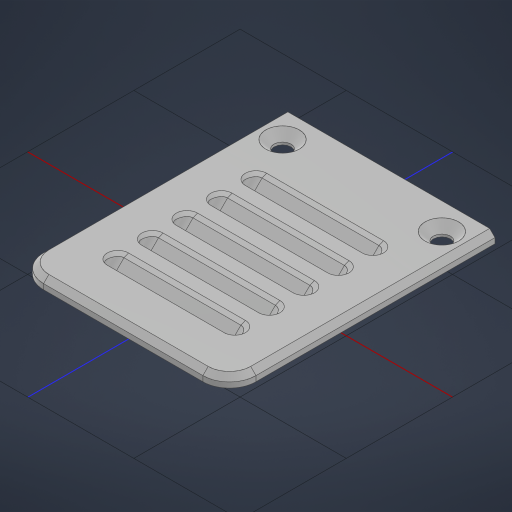
# Autodesk Inventor part: LED-Ring_Camera-Cover
Saved by Autodesk Inventor 2023.2 (Build 272271030, 271C)
## iProperties
Created: 2023-02-19
Part Number: LED-Ring_Camera-Cover
Material: Generisch
Document SubType Name: Modeling
Designer: Stefan
Mass: 3.244 g
Surface Area: 44.6567 cm^2
Volume: 3.244 cm^3
Density: 1 g/cm^3
Appearance: Glatt - Mittelgrau
Author: Stefan
Autodesk Inventor part; units mm, degrees
ref_plane "YZ Plane" through (0, 0, 0) normal (1, 0, 0) x (0, 1, 0)
ref_plane "XZ Plane" through (0, 0, 0) normal (0, 1, 0) x (-1, 0, 0)
ref_plane "XY Plane" through (0, 0, 0) normal (0, 0, 1) x (1, 0, 0)
sketch "Skizze1" plane through (0, 0, 0) normal (0, 1, 0) x (-1, 0, 0)
  arc A0 (20, 17) -> (15, 22) centre (15, 17) ccw
  arc A1 (-15, 22) -> (-20, 17) centre (-15, 17) ccw
  line L0 (20, -40) -> (-20, -40) construction
  line L1 (-20, -40) -> (-20, 22) construction
  line L2 (-20, 22) -> (20, 22) construction
  line L3 (20, 22) -> (20, -40) construction
  line L4 (20, -40) -> (-20, -40)
  line L5 (15, 22) -> (-15, 22)
  line L6 (20, -40) -> (20, 17)
  line L7 (-20, 17) -> (-20, -40)
  line L8 (0, -40) -> (0, 22) construction
  arc A2 (18, 17) -> (15, 20) centre (15, 17) ccw construction
  arc A3 (-15, 20) -> (-18, 17) centre (-15, 17) ccw construction
  line L9 (-15, 20) -> (15, 20) construction
  line L10 (20, -28) -> (-20, -28)
  line L11 (-20, -28) -> (-20, -26)
  line L12 (20, -26) -> (20, -28)
  circle A4 centre (-15, -23) radius 5 construction
  circle A5 centre (15, -23) radius 5 construction
  line L13 (-18, -18) -> (-15, -18) construction
  line L14 (-10, -23) -> (-10, -26) construction
  line L15 (15, -18) -> (18, -18) construction
  line L16 (10, -23) -> (10, -26) construction
  arc A6 (-10, -23) -> (-15, -18) centre (-15, -23) ccw construction
  arc A7 (15, -18) -> (10, -23) centre (15, -23) ccw construction
  circle A8 centre (-15, -23) radius 2.25
  circle A9 centre (15, -23) radius 2.25
  line L17 (-11, 14) -> (11, 14) construction
  line L18 (-11, 12.5) -> (11, 12.5)
  line L19 (11, 15.5) -> (-11, 15.5)
  arc A10 (-11, 15.5) -> (-11, 12.5) centre (-11, 14) ccw
  arc A11 (11, 12.5) -> (11, 15.5) centre (11, 14) ccw
  line L20 (18, 17) -> (18, -18) construction
  line L21 (-18, -18) -> (-18, 17) construction
  line L22 (10, -26) -> (-10, -26) construction
  line L23 (-9.9, -25.9) -> (-9.9, -23)
  arc A12 (-9.9, -23) -> (-15, -17.9) centre (-15, -23) ccw
  line L24 (-15, -17.9) -> (-17.9, -17.9)
  line L25 (-17.9, -17.9) -> (-17.9, 17)
  arc A13 (-15, 19.9) -> (-17.9, 17) centre (-15, 17) ccw
  line L26 (-15, 19.9) -> (15, 19.9)
  arc A14 (17.9, 17) -> (15, 19.9) centre (15, 17) ccw
  line L27 (17.9, 17) -> (17.9, -17.9)
  line L28 (17.9, -17.9) -> (15, -17.9)
  arc A15 (15, -17.9) -> (9.9, -23) centre (15, -23) ccw
  line L29 (9.9, -23) -> (9.9, -25.9)
  line L30 (9.9, -25.9) -> (-9.9, -25.9)
  line L31 (-8.9, -24.9) -> (-8.9, -23)
  arc A16 (-8.9, -23) -> (-15, -16.9) centre (-15, -23) ccw
  line L32 (-15, -16.9) -> (-16.9, -16.9)
  line L33 (-16.9, -16.9) -> (-16.9, 17)
  arc A17 (-15, 18.9) -> (-16.9, 17) centre (-15, 17) ccw
  line L34 (-15, 18.9) -> (15, 18.9)
  arc A18 (16.9, 17) -> (15, 18.9) centre (15, 17) ccw
  line L35 (16.9, 17) -> (16.9, -16.9)
  line L36 (16.9, -16.9) -> (15, -16.9)
  arc A19 (15, -16.9) -> (8.9, -23) centre (15, -23) ccw
  line L37 (8.9, -23) -> (8.9, -24.9)
  line L38 (8.9, -24.9) -> (-8.9, -24.9)
  point P0 (0, 0)
  point P1 (0, 0)
  point P2 (0, 0)
  point P3 (0, 20)
  point P4 (0, -26)
  point P5 (-20, -28)
  point P6 (-15.65, -19.3)
  point P7 (0, 14)
  dimension "d3" = 40
  dimension "d7" = 5
  dimension "d41" = 12
  dimension "d42" = 2
  dimension "d43" = 2
  dimension "d49" = 22
  dimension "d50" = 3
  dimension "d51" = 25
  dimension "d64" = 2
  dimension "d65" = 26
  dimension "d66" = 0.1
  dimension "d67" = 1
  dimension "d80" = 8
  dimension "d123" = 10
  dimension "d124" = 4.5
  constraints: 80 end point, 36 point on circle, 20 centre point, 18 tangent, 15 perpendicular, 8 parallel, 8 point on line, 5 coincident, 4 collinear, 3 equal radius, 3 midpoint, 2 horizontal, 23 other
  measures "d3" distance between parallel lines of L1 L3
  measures "d7" radius of A0
  measures "d41" distance between parallel lines of L0 L10
  measures "d42" radial gap between concentric circles of A3 A1
  measures "d43" radial gap between concentric circles of A2 A0
  measures "d49" distance from line of point (0, 0) L2
  measures "d50" diameter of A11
  measures "d64" distance between parallel lines of L10 L22
  measures "d65" distance from line of point (0, 0) L22
  measures "d66" distance between parallel lines of L22 L30
  measures "d67" distance between parallel lines of L30 L38
  measures "d80" distance between parallel lines of L17 L5
  measures "d123" diameter of A4
  measures "d124" diameter of A8
extrude "Extrusion1" add sketch "Skizze1" along normal blind 2 contours L6 L10 L7 A1 L5 A0 | A8 | A9 | A10 L19 A11 L18 | L23 A12 L24 L25 A13 L26 A14 L27 L28 A15 L29 L30 | L31 A16 L32 L33 A17 L34 A18 L35 L36 A19 L37 L38
extrude "Extrusion7" add sketch "Skizze1" against normal blind 1 contours L23 A12 L24 L25 A13 L26 A14 L27 L28 A15 L29 L30
sketch "Skizze5" plane through (0, 2, 0) normal (0, 1, 0) x (1, 0, 0)
  arc A0 (-20, -17) -> (-15, -22) centre (-15, -17) ccw projected
  line L0 (-15, -22) -> (15, -22) projected
  arc A1 (15, -22) -> (20, -17) centre (15, -17) ccw projected
  line L1 (20, -17) -> (20, 28) projected
  line L2 (20, 28) -> (-20, 28) projected
  line L3 (-20, 28) -> (-20, -17) projected
  line L4 (-15, -22) -> (15, -22) projected
  line L5 (0, -22) -> (0, 28) construction
  line L6 (20, 28) -> (-20, 28) projected
  line L7 (11, -12) -> (-11, -12) construction
  line L8 (11, -10.5) -> (-11, -10.5)
  line L9 (-11, -13.5) -> (11, -13.5)
  arc A2 (11, -13.5) -> (11, -10.5) centre (11, -12) ccw
  arc A3 (-11, -10.5) -> (-11, -13.5) centre (-11, -12) ccw
  circle A4 centre (15, 23) radius 5 construction
  circle A5 centre (-15, 23) radius 5 construction
  line L10 (20, -17) -> (20, 28) projected
  line L11 (-20, 28) -> (-20, -17) projected
  point P0 (0, 0)
  point P1 (0, -12)
  dimension "d70" = 3
  dimension "d71" = 25
  dimension "d72" = 10
  dimension "d115" = 10
  constraints: 10 end point, 8 tangent, 4 centre point, 4 point on circle, 3 midpoint, 1 equal radius, 1 parallel, 1 perpendicular, 1 point on line
  measures "d70" diameter of A3
  measures "d72" distance between parallel lines of L7 L0
  measures "d115" diameter of A4
loft "Erhebung1" cut profiles "Skizze5", "Skizze1" contours A2 L9 A3 L8 / A10 L19 A11 L18
pattern_linear "Rechteckige Anordnung1" count 5 spacing 6.5 along (0, 0, -1) of "Erhebung1"
hole "Bohrung3" at (15, 2, -23) at (-15, 2, -23) direction (0, -1, 0) diameter 3.2 end through all countersink diameter 6.3 countersink angle 90 clearance for "Flachkopfsenkschraube ISO 2009/7046" size "M3" standard "ISO"
chamfer "Fase1" distance 1 angle 45 5 edges at (20, 2, -5.5) (18.5355, 2, 20.5355) (0, 2, 22) (-18.5355, 2, 20.5355) (-20, 2, -5.5)
chamfer "Fase2" distance 0.5 angle 45 20 edges at (12.5, 2, 12) (0, 2, 13.5) (-12.5, 2, 12) (0, 2, 10.5) (12.5, 2, 5.5) (0, 2, 7) (-12.5, 2, 5.5) (0, 2, 4) (12.5, 2, -1) (0, 2, 0.5) (-12.5, 2, -1) (0, 2, -2.5) (12.5, 2, -7.5) (0, 2, -6) (-12.5, 2, -7.5) (0, 2, -9) (0, 2, -12.5) (-12.5, 2, -14) (0, 2, -15.5) (12.5, 2, -14)
equation "\"d42\" = d62"
equation "\"d43\" = d62"
equation "\"d62\" = 2"
